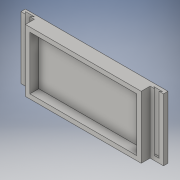
# Autodesk Inventor part: doveTailSide
Saved by Autodesk Inventor 2016 (Build 200138000, 138)
## iProperties
Created: 2015-11-04
Part Number: doveTailSide
Material: Generic
Document SubType Name: Modeling
Designer: rossmosier
Density: 1 g/cm^3
Appearance: Default
Author: rossmosier
Autodesk Inventor part; units mm, degrees
ref_plane "YZ Plane" through (0, 0, 0) normal (1, 0, 0) x (0, 1, 0)
ref_plane "XZ Plane" through (0, 0, 0) normal (0, 1, 0) x (-1, 0, 0)
ref_plane "XY Plane" through (0, 0, 0) normal (0, 0, 1) x (1, 0, 0)
sketch "Sketch2" plane through (0, 0, 0) normal (0, 0, 1) x (1, 0, 0)
  line L0 (0, 0) -> (203.2, 0)
  line L1 (203.2, 0) -> (203.2, 88.9)
  line L2 (203.2, 88.9) -> (0, 88.9)
  line L3 (0, 88.9) -> (0, 0)
  dimension "d6" = 203.2
  dimension "d7" = 88.9
  constraints: 8 end point, 2 parallel, 1 horizontal, 1 perpendicular
  measures "d6" distance of L2.end L1.end
  measures "d7" distance of L1.end L0.end
extrude "Extrusion2" add sketch "Sketch2" along normal blind 6.35
sketch "Sketch3" plane through (0, 0, 6.35) normal (0, 0, 1) x (1, 0, 0)
  line L0 (0, 0) -> (203.2, 0) projected
  line L1 (203.2, 0) -> (203.2, 88.9) projected
  line L2 (203.2, 88.9) -> (0, 88.9) projected
  line L3 (0, 88.9) -> (0, 0) projected
  line L4 (203.2, 88.9) -> (0, 88.9) construction
  line L5 (0, 0) -> (203.2, 0) construction
  line L6 (0, 88.9) -> (203.2, 0) construction
  line L7 (203.2, 0) -> (203.2, 88.9) construction
  line L8 (203.2, 88.9) -> (0, 0) construction
  line L9 (25.4, 6.35) -> (177.8, 6.35)
  line L10 (177.8, 6.35) -> (177.8, 82.55)
  line L11 (177.8, 82.55) -> (25.4, 82.55)
  line L12 (25.4, 82.55) -> (25.4, 6.35)
  line L13 (25.4, 6.35) -> (177.8, 82.55) construction
  line L14 (177.8, 6.35) -> (25.4, 82.55) construction
  line L15 (19.05, 88.9) -> (184.15, 88.9)
  line L16 (184.15, 88.9) -> (184.15, 0)
  line L17 (184.15, 0) -> (19.05, 0)
  line L18 (19.05, 0) -> (19.05, 88.9)
  point P0 (101.6, 44.45)
  dimension "d10" = 152.4
  dimension "d11" = 76.2
  dimension "d12" = 6.35
  constraints: 24 end point, 4 parallel, 3 midpoint, 2 perpendicular, 1 horizontal, 3 other
  measures "d10" distance of L11.end L10.end
  measures "d11" distance of L10.end L9.end
  measures "d12" distance between parallel lines of L11 L15
extrude "Extrusion3" add sketch "Sketch3" along normal blind 12.7 contours L18 L2 L16 L0
sketch "Sketch5" plane through (0, 88.9, 0) normal (0, 1, 0) x (1, 0, 0)
  line L0 (203.2, 0) -> (0, 0) projected
  line L1 (0, 0) -> (0, -6.35) projected
  line L2 (19.05, -6.35) -> (0, -6.35) projected
  line L3 (19.05, -6.35) -> (19.05, -19.05) projected
  line L4 (184.15, -19.05) -> (19.05, -19.05) projected
  line L5 (184.15, -6.35) -> (184.15, -19.05) projected
  line L6 (203.2, -6.35) -> (184.15, -6.35) projected
  line L7 (203.2, 0) -> (203.2, -6.35) projected
  line L8 (0, 0) -> (203.2, 0) construction
  line L9 (0, -6.35) -> (19.05, -6.35)
  line L10 (19.05, -6.35) -> (19.05, 0) construction
  line L11 (19.05, 0) -> (0, 0) construction
  line L12 (0, 0) -> (0, -6.35) construction
  line L13 (19.05, -6.35) -> (0, -6.35) construction
  line L14 (9.525, -6.35) -> (9.525, -3.175) construction
  line L15 (9.525, -6.35) -> (12.7, -6.35) construction
  line L16 (9.525, -6.35) -> (6.35, -6.35)
  line L17 (9.525, -3.175) -> (15.875, -3.175)
  line L18 (9.525, -3.175) -> (3.175, -3.175)
  line L19 (3.175, -3.175) -> (6.35, -6.35)
  line L20 (15.875, -3.175) -> (12.7, -6.35)
  line L21 (6.35, -6.35) -> (12.7, -6.35)
  line L22 (193.675, 0) -> (193.675, -6.35) construction
  line L23 (193.675, -6.35) -> (196.85, -6.35)
  line L24 (184.15, -6.35) -> (203.2, -6.35) projected
  line L25 (193.675, -6.35) -> (190.5, -6.35)
  line L26 (193.675, -4.2254) -> (187.325, -4.2254)
  line L27 (193.675, -4.2254) -> (200.025, -4.2254)
  line L28 (200.025, -4.2254) -> (196.85, -6.35)
  line L29 (187.325, -4.2254) -> (190.5, -6.35)
  dimension "d15" = 3.175
  dimension "d16" = 3.175
  dimension "d17" = 6.35
  dimension "d18" = 6.35
  dimension "d19" = 3.175
  dimension "d20" = 3.175
  dimension "d21" = 6.35
  dimension "d22" = 6.35
  constraints: 38 end point, 8 point on line, 5 horizontal, 2 midpoint, 2 parallel, 2 perpendicular, 1 collinear, 1 vertical
  measures "d15" distance of L14.start L15.end
  measures "d16" distance of L14.start L16.end
  measures "d17" distance of L14.end L17.end
  measures "d18" distance of L14.end L18.end
  measures "d19" distance of L22.end L23.end
  measures "d20" distance of L22.end L25.end
  measures "d21" distance of L26.start L26.end
  measures "d22" distance of L26.start L27.end
extrude "Extrusion4" cut sketch "Sketch5" against normal blind 82.55 contours L6 L29 L26 L27 L28 | L19 L18 L17 L20 L2
body "Solid2"
